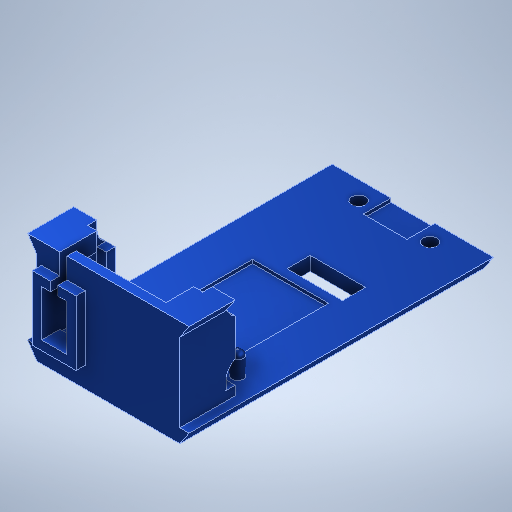
# Autodesk Inventor part: CarcazaV2
Saved by Autodesk Inventor 2025.1 (Build 291241020, 241B)
## iProperties
Created: 2024-08-30
Part Number: CarcazaV2
Material: Generic
Document SubType Name: Modeling
Designer: andre
Density: 1 g/cm^3
Appearance: Anodized - Blue
Author: andre
Autodesk Inventor part; units mm, degrees
ref_plane "YZ Plane" through (0, 0, 0) normal (1, 0, 0) x (0, 1, 0)
ref_plane "XZ Plane" through (0, 0, 0) normal (0, 1, 0) x (-1, 0, 0)
ref_plane "XY Plane" through (0, 0, 0) normal (0, 0, 1) x (1, 0, 0)
sketch "Sketch1" plane through (0, 0, 0) normal (0, 1, 0) x (-1, 0, 0)
  line L0 (0, 0) -> (31, 0)
  line L1 (31, 0) -> (31, -60)
  line L2 (31, -60) -> (0, -60)
  line L3 (0, -60) -> (0, 0)
  dimension "d0" = 31
  dimension "d1" = 60
  constraints: 8 end point, 2 parallel, 1 horizontal, 1 perpendicular
  measures "d0" distance of L0.start L0.end
  measures "d1" distance of L0.end L1.end
extrude "Extrusion1" add sketch "Sketch1" along normal blind 3
sketch "Sketch2" plane through (0, 3, 0) normal (0, 1, 0) x (1, 0, 0)
  line L0 (0, 60) -> (-31, 60) projected
  line L1 (-31, 60) -> (-31, 0) projected
  line L2 (-31, 0) -> (0, 0) projected
  line L3 (0, 0) -> (0, 60) projected
  line L4 (-23.75, 33.5) -> (-7.25, 33.5)
  line L5 (-7.25, 33.5) -> (-7.25, 14.5)
  line L6 (-7.25, 14.5) -> (-23.75, 14.5)
  line L7 (-23.75, 14.5) -> (-23.75, 33.5)
  line L8 (-23.75, 14.5) -> (-7.25, 33.5) construction
  line L9 (-23.75, 33.5) -> (-7.25, 14.5) construction
  line L10 (-20.25, 60) -> (-10.75, 60) construction
  line L11 (-10.75, 60) -> (-10.75, 54)
  line L12 (-10.75, 54) -> (-20.25, 54)
  line L13 (-20.25, 54) -> (-20.25, 60)
  point P0 (-15.5, 24)
  point P1 (-15.5, 24)
  point P2 (-15.5, 54)
  point P3 (-10.75, 57)
  point P4 (-15.5, 33.5)
  point P5 (-15.5, 14.5)
  point P6 (-15.5, 0)
  dimension "d4" = 16.5
  dimension "d5" = 19
  dimension "d8" = 6
  dimension "d9" = 9.5
  dimension "d32" = 39.5
  constraints: 20 end point, 7 midpoint, 4 parallel, 2 horizontal, 2 perpendicular, 2 vertical alignment, 1 point on line
  measures "d4" distance of L5.end L6.end
  measures "d5" distance of L4.end L5.end
  measures "d8" distance of L12.end L10.start
  measures "d9" distance of L11.end L12.end
  measures "d32" distance between parallel lines of L12 L6
extrude "Extrusion2" cut sketch "Sketch2" against normal blind 0.8 contours L11 L12 L13 L0 | L4 L5 L6 L7
sketch "Sketch10" plane through (0, 0, 0) normal (0, -1, 0) x (1, 0, 0)
  line L0 (-6.25, -40.5) -> (-18.25, -40.5)
  line L1 (-18.25, -40.5) -> (-18.25, -35.5)
  line L2 (-18.25, -35.5) -> (-6.25, -35.5)
  line L3 (-6.25, -35.5) -> (-6.25, -40.5)
  line L4 (-23.75, -33.5) -> (-7.25, -33.5) projected
  line L5 (-7.25, -33.5) -> (-7.25, -14.5) projected
  point P0 (0, 0)
  dimension "d36" = 12
  dimension "d37" = 5
  dimension "d38" = 7
  dimension "d39" = 1
  constraints: 8 end point, 2 parallel, 1 horizontal, 1 perpendicular
  measures "d36" distance of L0.start L0.end
  measures "d37" distance of L2.end L0.start
  measures "d38" distance between parallel lines of L4 L0
  measures "d39" distance between parallel lines of L3 L5
extrude "Extrusion7" cut sketch "Sketch10" against normal blind 10
sketch "Sketch11" plane through (0, 3, 0) normal (0, 1, 0) x (1, 0, 0)
  line L0 (-31, 6) -> (0, 6)
  line L1 (0, 6) -> (0, 4)
  line L2 (0, 4) -> (-31, 4)
  line L3 (-31, 4) -> (-31, 6)
  line L4 (-18.25, 35.5) -> (-18.25, 40.5) projected
  line L5 (-18.25, 40.5) -> (-6.25, 40.5) projected
  line L6 (-6.25, 40.5) -> (-6.25, 35.5) projected
  line L7 (-6.25, 35.5) -> (-18.25, 35.5) projected
  line L8 (-10.75, 60) -> (-10.75, 54) projected
  line L9 (-10.75, 54) -> (-20.25, 54) projected
  line L10 (-20.25, 54) -> (-20.25, 60) projected
  line L11 (-20.25, 60) -> (-31, 60) projected
  line L12 (-31, 60) -> (-31, 0) projected
  line L13 (-31, 0) -> (0, 0) projected
  line L14 (0, 0) -> (0, 60) projected
  line L15 (0, 60) -> (-10.75, 60) projected
  line L16 (-7.25, 33.5) -> (-7.25, 14.5) projected
  line L17 (-7.25, 14.5) -> (-23.75, 14.5) projected
  line L18 (-23.75, 14.5) -> (-23.75, 33.5) projected
  line L19 (-23.75, 33.5) -> (-7.25, 33.5) projected
  dimension "d42" = 8.5
  dimension "d43" = 2
  constraints: 8 end point, 2 parallel, 2 vertical alignment, 1 horizontal, 1 perpendicular
  measures "d42" distance between parallel lines of L17 L0
  measures "d43" distance between parallel lines of L0 L2
extrude "Extrusion8" add sketch "Sketch11" along normal blind 2 contours L0 L1 L2 L3
sketch "Sketch12" plane through (0, 3, 0) normal (0, 1, 0) x (1, 0, 0)
  line L0 (0, 4) -> (-31, 4) projected
  line L1 (-31, 4) -> (-31, 0) projected
  line L2 (-31, 0) -> (0, 0) projected
  line L3 (0, 0) -> (0, 4) projected
  line L4 (-31, 0) -> (0, 0) projected
  line L5 (-28, 0) -> (-3, 0)
  line L6 (-3, 0) -> (-3, 4)
  line L7 (-3, 4) -> (-28, 4)
  line L8 (-28, 4) -> (-28, 0)
  point P0 (-15.5, 4)
  point P1 (-15.5, 0)
  point P2 (-28, 4)
  point P3 (-3, 4)
  dimension "d46" = 25
  constraints: 8 end point, 2 midpoint, 2 parallel, 1 horizontal, 1 horizontal alignment, 1 perpendicular, 1 point on line, 1 vertical alignment
  measures "d46" distance of L6.end L7.end
extrude "Extrusion9" cut sketch "Sketch12" against normal blind 1 contours L6 L2 L8 L0
sketch "Sketch17" plane through (0, 2, 0) normal (0, 1, 0) x (1, 0, 0)
  line L0 (-3, 0) -> (-28, 0) projected
  line L1 (-3, 4) -> (-3, 0) projected
  line L2 (-28, 4) -> (-3, 4) projected
  line L3 (-28, 0) -> (-28, 4) projected
  line L4 (-28, 0) -> (-3, 0)
  line L5 (-3, 0) -> (-3, 2)
  line L6 (-3, 2) -> (-28, 2)
  line L7 (-28, 2) -> (-28, 0)
  point P0 (0, 0)
  dimension "d57" = 2
  constraints: 8 end point, 2 parallel, 1 horizontal, 1 midpoint, 1 perpendicular
  measures "d57" distance between parallel lines of L6 L2
extrude "Extrusion13" add sketch "Sketch17" along normal up to surface (1 mm away) contours L0 L3 L6 L1
sketch "Sketch18" plane through (0, 3, 0) normal (0, 1, 0) x (1, 0, 0)
  line L0 (-28, 2) -> (-28, 4) projected
  line L1 (-28, 4) -> (-31, 4) projected
  line L2 (-31, 4) -> (-31, 0) projected
  line L3 (-31, 0) -> (0, 0) projected
  line L4 (0, 0) -> (0, 4) projected
  line L5 (0, 4) -> (-3, 4) projected
  line L6 (-3, 4) -> (-3, 2) projected
  line L7 (-28, 2) -> (-3, 2) projected
  line L8 (-28, 2) -> (-28, 0)
  line L9 (-3, 2) -> (-3, 0)
  constraints: 4 end point, 2 perpendicular, 2 point on line
extrude "Extrusion14" add sketch "Sketch18" along normal blind 20 contours L8 L3 L2 L1 L0 | L6 L5 L4 L3 L9
sketch "Sketch19" plane through (-31, 0, 0) normal (0, 0, 1) x (1, 0, 0)
  line L0 (0, 0) -> (0, 23) projected
  line L1 (0, 0) -> (31, 0) projected
  line L2 (31, 0) -> (31, 23) projected
  line L3 (28, 23) -> (31, 23) projected
  line L4 (28, 3) -> (28, 23) projected
  line L5 (3, 3) -> (28, 3) projected
  line L6 (3, 3) -> (3, 23) projected
  line L7 (0, 23) -> (3, 23) projected
extrude "Extrusion15" add sketch "Sketch19" along normal blind 4
sketch "Sketch20" plane through (-31, 0, 4) normal (0, 0, 1) x (1, 0, 0)
  line L0 (3, 23) -> (0, 23) projected
  line L1 (0, 23) -> (31, 23)
  line L2 (31, 23) -> (31, 0)
  line L3 (31, 0) -> (0, 0)
  line L4 (0, 0) -> (0, 23)
  constraints: 8 end point, 2 parallel, 1 horizontal, 1 perpendicular
extrude "Extrusion16" add sketch "Sketch20" along normal blind 2
sketch "Sketch21" plane through (-31, 0, 6) normal (0, 0, 1) x (1, 0, 0)
  line L0 (8.5, 16.5) -> (3, 16.5)
  line L1 (3, 16.5) -> (3, 6.5)
  line L2 (3, 6.5) -> (8.5, 6.5)
  line L3 (8.5, 6.5) -> (8.5, 16.5)
  line L4 (0, 23) -> (0, 0) projected
  line L5 (0, 0) -> (31, 0) projected
  point P0 (5.75, 6.5)
  dimension "d66" = 5.5
  dimension "d67" = 10
  dimension "d68" = 3
  dimension "d69" = 6.5
  constraints: 8 end point, 2 parallel, 1 horizontal, 1 midpoint, 1 perpendicular
  measures "d66" distance of L1.end L2.end
  measures "d67" distance of L2.end L0.start
  measures "d68" distance between parallel lines of L4 L1
  measures "d69" distance from line of point (5.75, 6.5) L5
extrude "Extrusion17" cut sketch "Sketch21" against normal blind 2
sketch "Sketch22" plane through (-31, 0, 6) normal (0, 0, 1) x (1, 0, 0)
  line L0 (8.5, 6.5) -> (3, 6.5) projected
  line L1 (3, 6.5) -> (3, 16.5) projected
  line L2 (3, 16.5) -> (8.5, 16.5) projected
  line L3 (8.5, 16.5) -> (8.5, 6.5) projected
  line L4 (0, 0) -> (31, 0) projected
  line L5 (31, 0) -> (31, 23) projected
  line L6 (31, 23) -> (0, 23) projected
  line L7 (0, 23) -> (0, 0) projected
  line L8 (10.5, 18.5) -> (1, 18.5)
  line L9 (1, 18.5) -> (1, 4.5)
  line L10 (1, 4.5) -> (10.5, 4.5)
  line L11 (10.5, 4.5) -> (10.5, 18.5)
  dimension "d72" = 2
  constraints: 8 end point, 3 other
  measures "d72" distance between parallel lines of L2 L8
extrude "Extrusion18" add sketch "Sketch22" along normal blind 2 contours L11 L10 L9 L8
sketch "Sketch24" plane through (0, 5, -4) normal (0, 0, -1) x (-1, 0, 0)
  line L0 (0, 0) -> (0, 18) projected
  line L1 (0, 13) -> (5, 13)
  line L2 (5, 13) -> (5, 5)
  line L3 (5, 5) -> (0, 5)
  line L4 (0, 5) -> (0, 13)
  line L5 (3, 0) -> (3, 18) projected
  point P0 (0, -5)
  point P1 (5, 9)
  point P2 (0, 9)
  point P3 (0, 5)
  dimension "d75" = 2
  dimension "d76" = 8
  constraints: 8 end point, 2 midpoint, 2 parallel, 1 horizontal, 1 horizontal alignment, 1 perpendicular, 1 point on line
  measures "d75" distance between parallel lines of L5 L2
  measures "d76" distance between parallel lines of L3 L1
extrude "Extrusion19" add sketch "Sketch24" along normal blind 2
ref_plane "Work Plane1" through (-15.5, 0, -60) normal (1, 0, 0) x (0, 0, -1)
mirror "Mirror1" about plane through (-15.5, 0, -60) normal (1, 0, 0) of "Extrusion19"
sketch "Sketch25" plane through (0, 23, 0) normal (0, 1, 0) x (1, 0, 0)
  line L0 (-22.5, -8) -> (-22.5, -4) projected
  line L1 (-28, -4) -> (-22.5, -4) projected
  line L2 (-28, -4) -> (-28, -8) projected
  line L3 (-22.5, -8) -> (-28, -8) projected
  line L4 (-26, -4) -> (-24.5, -4)
  line L5 (-24.5, -4) -> (-24.5, -8)
  line L6 (-24.5, -8) -> (-26, -8)
  line L7 (-26, -8) -> (-26, -4)
  point P0 (0, 0)
  point P1 (-25.25, -4)
  point P2 (-25.25, -8)
  dimension "d79" = 1.5
  constraints: 8 end point, 2 midpoint, 2 parallel, 1 horizontal, 1 horizontal alignment, 1 perpendicular, 1 point on line, 1 vertical alignment
  measures "d79" distance between parallel lines of L5 L7
extrude "Extrusion20" cut sketch "Sketch25" against normal up to surface (16.5 mm away) contours L3 L7 L1 L5
fillet "Fillet1" radius 3.5875 4 edges at (-1.5, 18, -4) (-1.5, 10, -4) (-29.5, 18, -4) (-29.5, 10, -4)
sketch "Sketch26" plane through (-3, 2, -2) normal (0, 0, -1) x (-1, 0, 0)
  line L0 (25, 21) -> (22.3342, 21)
  line L1 (22.3342, 21) -> (22.3342, 17)
  line L2 (22.3342, 17) -> (25, 17)
  line L3 (25, 17) -> (25, 21)
  line L4 (25, 1) -> (23, 1)
  line L5 (23, 1) -> (23, 4)
  line L6 (23, 4) -> (25, 4)
  line L7 (25, 4) -> (25, 1)
  line L8 (25, 1) -> (0, 1) projected
  line L9 (0, 0) -> (0, 1) projected
  line L10 (25, 0) -> (0, 0) projected
  line L11 (25, 1) -> (25, 0) projected
  line L12 (23, 21) -> (23, 14.5) projected
  line L13 (23, 14.5) -> (25, 14.5) projected
  line L14 (25, 14.5) -> (25, 21) projected
  line L15 (23, 21) -> (25, 21) projected
  point P0 (-3, -2)
  point P1 (23, 8)
  point P2 (23, 17)
  dimension "d84" = 3
  dimension "d85" = 4
  constraints: 16 end point, 4 parallel, 2 horizontal, 2 horizontal alignment, 2 perpendicular, 2 vertical alignment, 1 coincident
  measures "d84" distance of L4.end L5.end
  measures "d85" distance of L0.end L1.end
extrude "Extrusion21" add sketch "Sketch26" against normal up to surface (6 mm away) contours L3 L2 L12 L0 | L4 L5 L6 L7
mirror "Mirror2" about plane through (-15.5, 0, -60) normal (1, 0, 0) of "Extrusion21"
sketch "Sketch27" plane through (0, 0, 0) normal (0, -1, 0) x (1, 0, 0)
  line L0 (-10.75, -60) -> (-10.75, -54) projected
  line L1 (-20.25, -60) -> (-10.75, -60) projected
  line L2 (-20.25, -54) -> (-20.25, -60) projected
  line L3 (-10.75, -54) -> (-20.25, -54) projected
  circle A0 centre (-7.75, -56) radius 1.5
  circle A1 centre (-23.25, -56) radius 1.5
  line L4 (0, -60) -> (-31, -60) projected
  point P0 (0, 0)
  dimension "d88" = 3
  dimension "d89" = 3
  dimension "d90" = 4
  dimension "d91" = 3
  constraints: 2 centre point, 1 equal radius, 1 horizontal alignment
  measures "d88" distance from line of L2 A1.centre
  measures "d89" distance from line of L0 A0.centre
  measures "d90" distance from line of L4 A0.centre
  measures "d91" diameter of A0
extrude "Extrusion22" cut sketch "Sketch27" against normal through all contours A0 | A1
sketch "Sketch28" plane through (0, 3, 0) normal (0, 1, 0) x (1, 0, 0)
  circle A0 centre (-7.75, 56) radius 1.5 projected
  circle A1 centre (-23.25, 56) radius 1.5 projected
  line L0 (-31, 6) -> (0, 6) projected
  line L1 (0, 6) -> (0, 60) projected
  line L2 (0, 60) -> (-10.75, 60) projected
  line L3 (-10.75, 60) -> (-10.75, 54) projected
  line L4 (-10.75, 54) -> (-20.25, 54) projected
  line L5 (-20.25, 54) -> (-20.25, 60) projected
  line L6 (-20.25, 60) -> (-31, 60) projected
  line L7 (-31, 60) -> (-31, 6) projected
  line L8 (-18.25, 35.5) -> (-18.25, 40.5) projected
  line L9 (-18.25, 40.5) -> (-6.25, 40.5) projected
  line L10 (-6.25, 40.5) -> (-6.25, 35.5) projected
  line L11 (-6.25, 35.5) -> (-18.25, 35.5) projected
  line L12 (-7.25, 33.5) -> (-7.25, 14.5) projected
  line L13 (-7.25, 14.5) -> (-23.75, 14.5) projected
  line L14 (-23.75, 14.5) -> (-23.75, 33.5) projected
  line L15 (-23.75, 33.5) -> (-7.25, 33.5) projected
  line L16 (-7.25, 14.5) -> (-23.75, 14.5) projected
  line L17 (-7.25, 33.5) -> (-7.25, 14.5) projected
  line L18 (-23.75, 33.5) -> (-7.25, 33.5) projected
  line L19 (-23.75, 14.5) -> (-23.75, 33.5) projected
  circle A2 centre (-27.5, 10) radius 1.25
  circle A3 centre (-3.5, 10) radius 1.25
  point P0 (0, 0)
  dimension "d94" = 2.5
  dimension "d95" = 4.5
  dimension "d97" = 3.75
  dimension "d101" = 3.75
  constraints: 2 centre point, 1 equal radius, 1 horizontal alignment
  measures "d94" diameter of A2
  measures "d95" distance from line of L13 A2.centre
  measures "d97" distance from line of A2.centre L14
  measures "d101" distance from line of L12 A3.centre
extrude "Extrusion23" add sketch "Sketch28" along normal blind 5 contours A2 | A3
fillet "Fillet2" radius 1.1 2 edges at (-28.75, 8, -10) (-4.75, 8, -10)
sketch "Sketch29" plane through (0, 0, -60) normal (0, 0, -1) x (-1, 0, 0)
  line L0 (0, 3) -> (-2, 3)
  line L1 (-2, 3) -> (0, 0)
  line L2 (31, 3) -> (33, 3)
  line L3 (33, 3) -> (31, 0)
  line L4 (28, 2) -> (3, 2) projected
  line L5 (10.75, 2.2) -> (10.75, 3) projected
  line L6 (0, 3) -> (10.75, 3) projected
  line L7 (0, 0) -> (0, 3) projected
  line L8 (0, 0) -> (31, 0) projected
  line L9 (31, 0) -> (31, 3) projected
  line L10 (20.25, 3) -> (31, 3) projected
  line L11 (20.25, 3) -> (20.25, 2.2) projected
  line L12 (20.25, 2.2) -> (10.75, 2.2) projected
  dimension "d102" = 2
  dimension "d103" = 2
  constraints: 8 end point, 2 horizontal
  measures "d102" distance of L0.start L0.end
  measures "d103" distance of L2.start L2.end
extrude "Extrusion24" add sketch "Sketch29" against normal up to surface (66 mm away) contours L7 L1 L0 | L9 L2 L3
sketch "Sketch30" plane through (-31, 0, 6) normal (0, 0, 1) x (1, 0, 0)
  line L0 (6.5, 23) -> (6.5, 18.5) projected
  line L1 (6.5, 18.5) -> (10.5, 18.5) projected
  line L2 (10.5, 18.5) -> (10.5, 4.5) projected
  line L3 (10.5, 4.5) -> (1, 4.5) projected
  line L4 (1, 4.5) -> (1, 18.5) projected
  line L5 (1, 18.5) -> (5, 18.5) projected
  line L6 (5, 18.5) -> (5, 23) projected
  line L7 (5, 23) -> (0, 23) projected
  line L8 (0, 23) -> (0, 3) projected
  line L9 (-2, 3) -> (0, 3) projected
  line L10 (0, 0) -> (-2, 3) projected
  line L11 (0, 0) -> (31, 0) projected
  line L12 (33, 3) -> (31, 0) projected
  line L13 (31, 3) -> (33, 3) projected
  line L14 (31, 3) -> (31, 23) projected
  line L15 (31, 23) -> (6.5, 23) projected
  line L16 (31, 23) -> (33, 23)
  line L17 (33, 23) -> (31, 20)
  line L18 (31, 3) -> (31, 23) projected
  line L19 (0, 23) -> (-2, 23)
  line L20 (-2, 23) -> (0, 20)
  line L21 (0, 23) -> (0, 3) projected
  point P0 (0, 20)
  dimension "d106" = 2
  dimension "d108" = 2
  dimension "d110" = 3
  dimension "d111" = 3
  constraints: 8 end point, 2 horizontal, 2 point on line
  measures "d106" distance of L14.end L16.end
  measures "d108" distance of L7.end L19.end
  measures "d110" distance of L14.end L17.end
  measures "d111" distance of L7.end L20.end
extrude "Extrusion25" add sketch "Sketch30" against normal blind 10 contours L16 L17 L14 | L8 L20 L19
fillet "Fillet3" radius 2 2 edges at (-28, 19, 1) (-3, 19, 1)
equation "\"w\" = 2"
body "Solid1"
